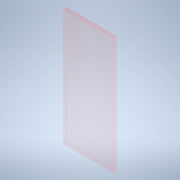
# Autodesk Inventor part: Placa
Saved by Autodesk Inventor 2021 (Build 250183000, 183)
## iProperties
Created: 2021-07-01
Part Number: Placa
Material: Acero inoxidable
Document SubType Name: Modeling
Designer: artur
Density: 8 g/cm^3
Appearance: Transparente - Rojo pulido
Mass: 4288.4 g
Surface Area: 1173.3 cm^2
Volume: 536.05 cm^3
Author: artur
Autodesk Inventor part; units mm, degrees
ref_plane "YZ Plane" through (0, 0, 0) normal (1, 0, 0) x (0, 1, 0)
ref_plane "XZ Plane" through (0, 0, 0) normal (0, 1, 0) x (-1, 0, 0)
ref_plane "XY Plane" through (0, 0, 0) normal (0, 0, 1) x (1, 0, 0)
sketch "Boceto1" plane through (0, 0, 0) normal (0, 0, 1) x (1, 0, 0)
  line L0 (0, 0) -> (151, 0)
  line L1 (151, 0) -> (151, 355)
  line L2 (151, 355) -> (0, 355)
  line L3 (0, 355) -> (0, 0)
  dimension "d0" = 151
  dimension "d1" = 355
  constraints: 8 end point, 2 parallel, 1 horizontal, 1 perpendicular
  measures "d0" distance of L1.end L2.end
  measures "d1" distance of L0.end L1.end
extrude "Extrusión1" add sketch "Boceto1" along normal blind 10
